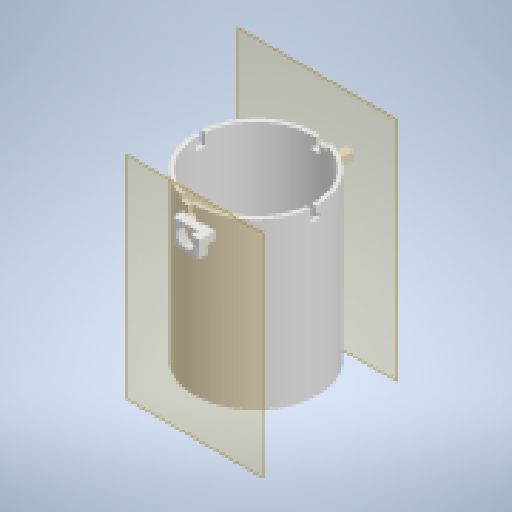
# Autodesk Inventor part: main_body
Saved by Autodesk Inventor 2024 (Build 280153000, 153)
## iProperties
Created: 2025-11-24
Part Number: main_body
Material: Generic
Document SubType Name: Modeling
Designer: Aidan
Density: 1 g/cm^3
Appearance: Default
Author: Aidan
Autodesk Inventor part; units mm, degrees
ref_plane "YZ Plane" through (0, 0, 0) normal (1, 0, 0) x (0, 1, 0)
ref_plane "XZ Plane" through (0, 0, 0) normal (0, 1, 0) x (-1, 0, 0)
sketch "Sketch1" plane through (0, 0, 0) normal (0, 1, 0) x (-1, 0, 0)
  circle A0 centre (0, 0) radius 75
  dimension "d0" = 150
  constraints: 1 centre point, 1 coincident
  measures "d0" diameter of A0
extrude "Extrusion1" add sketch "Sketch1" along normal blind 200
sketch "Sketch2" plane through (0, 200, 0) normal (0, 1, 0) x (1, 0, 0)
  circle A0 centre (0, 0) radius 75 projected
  circle A1 centre (0, 0) radius 70
  dimension "d3" = 5
  constraints: 1 centre point
  measures "d3" radial gap between concentric circles of A0 A1
extrude "Extrusion2" cut sketch "Sketch2" against normal blind 195 contours A1
ref_plane "Work Plane1" through (0, 0, -75) normal (0, 0, 1) x (1, 0, 0)
sketch "Sketch4" plane through (0, 0, -75) normal (0, 0, 1) x (1, 0, 0)
  line L0 (15, 185) -> (-15, 185)
  line L1 (-15, 185) -> (-15, 155)
  line L2 (-15, 155) -> (15, 155)
  line L3 (15, 155) -> (15, 185)
  line L4 (15, 185) -> (-15, 155) construction
  line L5 (-15, 185) -> (15, 155) construction
  line L6 (75, 200) -> (-75, 200) construction
  line L7 (0, 170) -> (0, 200) construction
  circle A0 centre (0, 170) radius 11.05
  point P0 (0, 0)
  dimension "d8" = 30
  dimension "d9" = 30
  dimension "d10" = 30
  dimension "d15" = 22.1
  constraints: 14 end point, 2 midpoint, 2 parallel, 1 centre point, 1 coincident, 1 horizontal, 1 perpendicular, 1 vertical
  measures "d8" distance of L2.end L1.end
  measures "d9" distance of L1.end L0.end
  measures "d10" distance of L7.start L7.end
  measures "d15" diameter of A0
extrude "Extrusion3" add sketch "Sketch4" along normal blind 3 and the other way blind 10
mirror "Mirror1" about plane through (0, 0, 0) normal (0, 0, 1) of "Extrusion3"
sketch "Sketch5" plane through (0, 0, 0) normal (0, -1, 0) x (1, 0, 0)
  line L0 (15, -4) -> (-15, -4)
  line L1 (-15, -4) -> (-15, 4)
  line L2 (-15, 4) -> (15, 4)
  line L3 (15, 4) -> (15, -4)
  line L4 (15, -4) -> (-15, 4) construction
  line L5 (-15, -4) -> (15, 4) construction
  circle A0 centre (0, 0) radius 75 projected
  dimension "d27" = 30
  dimension "d28" = 8
  constraints: 12 end point, 2 midpoint, 2 parallel, 1 coincident, 1 horizontal, 1 perpendicular
  measures "d27" distance of L1.end L2.end
  measures "d28" distance of L0.end L1.end
extrude "Extrusion4" add sketch "Sketch5" along normal blind 35 contours L0 L1 L2 L3
sketch "Sketch7" plane through (-15, 0, 4) normal (0, 0, 1) x (1, 0, 0)
  circle A0 centre (15, -20) radius 11.05
  line L0 (0, 0) -> (0, -35) projected
  line L1 (30, -35) -> (0, -35) projected
  point P0 (15, 0)
  dimension "d29" = 22.1
  dimension "d30" = 15
  dimension "d31" = 15
  constraints: 1 centre point
  measures "d29" diameter of A0
  measures "d30" distance from line of L0 A0.centre
  measures "d31" distance from line of L1 A0.centre
extrude "Extrusion6" cut sketch "Sketch7" against normal up to surface (8 mm away)
sketch "Sketch8" plane through (-15, 0, 4) normal (0, 0, 1) x (1, 0, 0)
  circle A0 centre (15, -20) radius 11.05 projected
  line L0 (0, 0) -> (30, 0) projected
  line L1 (0, 0) -> (0, -35) projected
  line L2 (30, -35) -> (0, -35) projected
  line L3 (30, 0) -> (30, -35) projected
  arc A1 (0, -20) -> (30, -20) centre (15, -18.2651) ccw
  line L4 (0, -20) -> (30, -20)
  line L5 (30, -20) -> (30, -35)
  line L6 (30, -35) -> (0, -35)
  line L7 (0, -35) -> (0, -20)
  dimension "d37" = 15.1
  constraints: 8 end point, 2 parallel, 2 point on circle, 2 point on line, 1 centre point, 1 horizontal, 1 midpoint, 1 perpendicular
  measures "d37" radius of A1
extrude "Extrusion8" cut sketch "Sketch8" against normal blind 35 contours L3 L2 L1 A1
sketch "Sketch9" plane through (15, 155, 73.4847) normal (1, 0, 0) x (0, 0, -1)
  line L0 (-11.5153, 30) -> (0, 30) projected
  line L1 (0, 30) -> (-20, 30)
  line L2 (-20, 30) -> (-20, 20)
  line L3 (-20, 20) -> (0, 20)
  line L4 (0, 20) -> (0, 30)
  point P0 (73.4847, -155)
  dimension "d40" = 20
  dimension "d41" = 10
  constraints: 8 end point, 2 parallel, 1 horizontal, 1 perpendicular
  measures "d40" distance of L3.end L2.end
  measures "d41" distance of L2.end L1.end
extrude "Extrusion9" add sketch "Sketch9" along normal blind 10
mirror "Mirror2" about plane through (0, 0, 0) normal (0, 0, 1) of "Extrusion9"
chamfer "Chamfer1" distance 3 angle 45 2 edges at (15, 175, 89.2423) (15, 175, -89.2423)
ref_plane "Work Plane2" through (0, 0, 75) normal (0, 0, 1) x (1, 0, 0)
sketch "Sketch10" plane through (0, 0, 75) normal (0, 0, 1) x (1, 0, 0)
  line L0 (2.6, 190.2) -> (-2.6, 190.2)
  line L1 (-2.6, 190.2) -> (-2.6, 185)
  line L2 (-2.6, 185) -> (2.6, 185)
  line L3 (2.6, 185) -> (2.6, 190.2)
  line L4 (-15, 155) -> (-15, 185) projected
  line L5 (15, 155) -> (-15, 155) projected
  line L6 (15, 175) -> (15, 155) projected
  line L7 (15, 175) -> (18, 175) projected
  line L8 (18, 175) -> (15, 178) projected
  line L9 (15, 185) -> (15, 178) projected
  line L10 (-15, 185) -> (15, 185) projected
  circle A0 centre (0, 170) radius 11.05 projected
  line L11 (15, 185) -> (-15, 185) construction
  line L12 (0, 185) -> (0, 170) construction
  line L13 (-70, 200) -> (70, 200) projected
  line L14 (-2.6, 185) -> (-7.8, 185)
  line L15 (-7.8, 185) -> (-7.8, 200)
  line L16 (-7.8, 200) -> (-2.6, 200)
  line L17 (-2.6, 200) -> (-2.6, 185)
  point P0 (0, 0)
  dimension "d50" = 5.2
  dimension "d51" = 5.2
  dimension "d52" = 5.2
  constraints: 18 end point, 4 parallel, 2 horizontal, 2 perpendicular, 1 collinear, 1 midpoint, 1 point on line, 1 vertical
  measures "d50" distance of L2.end L1.end
  measures "d51" distance of L1.end L0.end
  measures "d52" distance of L15.end L16.end
extrude "Extrusion10" cut sketch "Sketch10" against normal up to surface contours L3 L2 L1 L0 | L1 L10 L15 L13 L17
pattern_circular "Circular Pattern1" count 4 over 360 about axis through (0, 200, 0) along (0, -1, 0) of "Extrusion10"
sketch "Sketch11" plane through (0, 0, 75) normal (0, 0, 1) x (1, 0, 0)
  line L0 (-70, 5) -> (70, 5) projected
  line L1 (69.5641, 200) -> (69.5641, 185) projected
  line L2 (69.5641, 185) -> (69.9517, 185) projected
  line L3 (69.9517, 185) -> (69.9517, 190.2) projected
  line L4 (69.9517, 190.2) -> (69.9517, 190.2) projected
  line L5 (69.9517, 190.2) -> (69.9517, 200) projected
  line L6 (7.8, 200) -> (69.9517, 200) projected
  line L7 (7.8, 200) -> (7.8, 185) projected
  line L8 (7.8, 185) -> (-2.6, 185) projected
  line L9 (-2.6, 185) -> (-2.6, 190.2) projected
  line L10 (-2.6, 190.2) -> (2.6, 190.2) projected
  line L11 (2.6, 190.2) -> (2.6, 200) projected
  line L12 (-69.5641, 200) -> (2.6, 200) projected
  line L13 (-69.5641, 200) -> (-69.5641, 185) projected
  line L14 (-69.5641, 185) -> (-69.9517, 185) projected
  line L15 (-69.9517, 185) -> (-69.9517, 190.2) projected
  line L16 (-69.9517, 190.2) -> (-69.9517, 190.2) projected
  line L17 (-69.9517, 190.2) -> (-69.9517, 200) projected
  line L18 (-7.8, 200) -> (-69.9517, 200) projected
  line L19 (-7.8, 200) -> (-7.8, 185) projected
  line L20 (-7.8, 185) -> (2.6, 185) projected
  line L21 (2.6, 185) -> (2.6, 190.2) projected
  line L22 (2.6, 190.2) -> (-2.6, 190.2) projected
  line L23 (-2.6, 190.2) -> (-2.6, 200) projected
  line L24 (69.5641, 200) -> (-2.6, 200) projected
  line L25 (-17.8, 200) -> (-7.8, 200)
  line L26 (-7.8, 200) -> (-7.8, 195)
  line L27 (-7.8, 195) -> (-17.8, 195)
  line L28 (-17.8, 195) -> (-17.8, 200)
  point P0 (0, 0)
  dimension "d58" = 10
  dimension "d59" = 5
  constraints: 8 end point, 2 parallel, 1 collinear, 1 horizontal, 1 perpendicular, 1 point on line
  measures "d58" distance of L26.end L27.end
  measures "d59" distance of L25.end L26.end
extrude "Extrusion11" cut sketch "Sketch11" against normal up to surface contours L19 L27 L28 L12
pattern_circular "Circular Pattern2" count 2 over 360 about axis through (0, 0, 0) along (0, 1, 0) of "Extrusion11"
body "Solid1"
